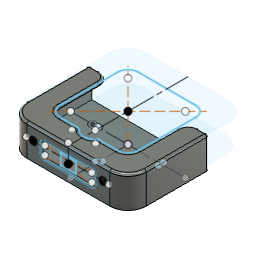
netgear-m5-wall-mount (Autodesk Fusion 360 design; units mm, degrees)
Autodesk Fusion 360 part; units mm, degrees
sketch "inner_space" plane through (0, 0, 0) normal (0, 1, 0) x (1, 0, 0)
  line L0 (-54.75, -54.75) -> (54.75, -54.75)
  line L1 (54.75, -54.75) -> (54.75, 54.75)
  line L2 (54.75, 54.75) -> (-54.75, 54.75)
  line L3 (-54.75, 54.75) -> (-54.75, -54.75)
  line L4 (-54.75, -54.75) -> (54.75, 54.75) construction
  line L5 (54.75, -54.75) -> (-54.75, 54.75) construction
  dimension "d21" = 109.5
  constraint horizontal L0
  constraint perpendicular L0 L1
  constraint parallel L0 L2
  constraint parallel L1 L3
  constraint coincident L4 origin
  constraint coincident L5 origin
  constraint equal L1 L2
  measures "d21" distance of L1.end L2.end
extrude "Extrude3" add sketch "inner_space" along normal blind 12.625 and the other way blind 12.625 makes body 1
fillet "Fillet2" radius 15 4 edges at (-54.75, 0, 54.75) (-54.75, 0, -54.75) (54.75, 0, 54.75) (54.75, 0, -54.75) on bodies 1
shell "Shell3" thickness 2.5 outward yes removed faces 0 bodies 1
sketch "bottom_ports" plane through (0, 0, 57.25) normal (0, 0, 1) x (1, 0, 0)
  line L0 (39.75, -15.125) -> (39.75, 15.125)
  line L1 (39.75, 15.125) -> (-39.75, 15.125)
  line L2 (-39.75, 15.125) -> (-39.75, -15.125)
  line L3 (-39.75, -15.125) -> (39.75, -15.125)
  line L4 (-7.2483, 5.7358) -> (7.2575, 5.7358)
  line L5 (7.2575, 5.7358) -> (7.2575, -4.8362)
  line L6 (7.2575, -4.8362) -> (-7.2483, -4.8362)
  line L7 (-7.2483, -4.8362) -> (-7.2483, 5.7358)
  line L8 (-40.1936, 2.575) -> (38.7277, 2.575) construction
  circle A0 centre (-33.5, 2.575) radius 3.3
  line L9 (0, 0) -> (0, 17.6954)
  circle A1 centre (33.5, 2.575) radius 3.3
  line L10 (22.5661, -8.0262) -> (-22.5661, -8.0262)
  line L11 (-26.5661, -4.0262) -> (-26.5661, 4.0262)
  line L12 (-22.5661, 8.0262) -> (22.5661, 8.0262)
  line L13 (26.5661, 4.0262) -> (26.5661, -4.0262)
  line L14 (26.5661, -8.0262) -> (-26.5661, 8.0262) construction
  line L15 (-26.5661, -8.0262) -> (26.5661, 8.0262) construction
  arc A2 (-22.5661, 8.0262) -> (-26.5661, 4.0262) centre (-22.5661, 4.0262) ccw
  arc A3 (-26.5661, -4.0262) -> (-22.5661, -8.0262) centre (-22.5661, -4.0262) ccw
  arc A4 (22.5661, -8.0262) -> (26.5661, -4.0262) centre (22.5661, -4.0262) ccw
  arc A5 (26.5661, 4.0262) -> (22.5661, 8.0262) centre (22.5661, 4.0262) ccw
  dimension "d41" = 6.6
  dimension "d45" = 4
  dimension "d91" = 33.5
  dimension "d94" = 17.7
  constraint horizontal L4
  constraint vertical L5
  constraint horizontal L6
  constraint vertical L7
  constraint perpendicular L0 L8
  constraint coincident L8 A0.centre
  constraint coincident L9.start origin
  constraint perpendicular L8 L9
  constraint symmetric A0 L9 A1
  constraint horizontal L10
  constraint perpendicular L10 L11
  constraint parallel L10 L12
  constraint parallel L11 L13
  constraint coincident L14 L9.start
  constraint coincident L15 L9.start
  constraint coincident L14.end L12
  constraint coincident L14.end L11
  constraint tangent L12 A2
  constraint tangent L11 A2
  constraint coincident L15.start L10
  constraint coincident L15.start L11
  constraint tangent L10 A3
  constraint tangent L11 A3
  constraint equal A2 A3
  constraint coincident L14.start L10
  constraint coincident L14.start L13
  constraint tangent L10 A4
  constraint tangent L13 A4
  constraint equal A2 A4
  constraint coincident L15.end L12
  constraint coincident L15.end L13
  constraint tangent L12 A5
  constraint tangent L13 A5
  constraint equal A2 A5
  measures "d41" diameter of A0
  measures "d45" radius of A2
  measures "d91" horizontal distance of A0.centre L9.end
  measures "d94" distance of L3 A0.centre
extrude "Extrude4" cut sketch "bottom_ports" against normal blind 10 contours L4 L5 L6 L7 | A0 | A1 | L10 L11 L12 L13 A2 A3 A4 A5 bodies 1
sketch "top_cutouts" plane through (0, 15.125, 0) normal (0, 1, 0) x (-1, 0, 0)
  arc A0 (-57.25, -39.75) -> (-39.75, -57.25) centre (-39.75, -39.75) ccw
  line L0 (-39.75, -57.25) -> (39.75, -57.25)
  arc A1 (39.75, -57.25) -> (57.25, -39.75) centre (39.75, -39.75) ccw
  line L1 (57.25, -39.75) -> (57.25, 39.75)
  arc A2 (57.25, 39.75) -> (39.75, 57.25) centre (39.75, 39.75) ccw
  line L2 (39.75, 57.25) -> (-39.75, 57.25)
  arc A3 (-39.75, 57.25) -> (-57.25, 39.75) centre (-39.75, 39.75) ccw
  line L3 (-57.25, 39.75) -> (-57.25, -39.75)
  line L4 (37.5, 27.5) -> (37.5, -27.5)
  line L5 (27.5, -37.5) -> (-27.5, -37.5)
  line L6 (-37.5, -27.5) -> (-37.5, 27.5)
  line L7 (-37.5, 37.5) -> (37.5, -37.5) construction
  line L8 (37.5, 37.5) -> (-37.5, -37.5) construction
  line L9 (0, -57.25) -> (0, 57.25)
  line L10 (-11.3811, 37.5) -> (-37.5, 37.5) construction
  line L11 (11.3811, 37.5) -> (27.5, 37.5)
  line L12 (-9.016, 37.5) -> (-27.5, 37.5)
  arc A4 (7.7879, 39.023) -> (-7.7879, 39.023) centre (0, 31.4868) ccw
  arc A5 (27.5, -37.5) -> (37.5, -27.5) centre (27.5, -27.5) ccw
  arc A6 (-37.5, -27.5) -> (-27.5, -37.5) centre (-27.5, -27.5) ccw
  arc A7 (-27.5, 37.5) -> (-37.5, 27.5) centre (-27.5, 27.5) ccw
  arc A8 (37.5, 27.5) -> (27.5, 37.5) centre (27.5, 27.5) ccw
  arc A9 (7.7879, 39.023) -> (11.3811, 37.5) centre (11.3811, 42.5) ccw
  arc A10 (-11.3811, 37.5) -> (-7.7879, 39.023) centre (-11.3811, 42.5) ccw
  dimension "d46" = 75
  dimension "d47" = 75
  dimension "d48" = 10
  dimension "d49" = 10
  dimension "d50" = 10
  dimension "d51" = 10
  dimension "d52" = 5
  dimension "d53" = 5
  constraint parallel L4 L6
  constraint coincident L7 origin
  constraint coincident L8 origin
  constraint midpoint L0 L9.start
  constraint midpoint L2 L9.end
  constraint perpendicular L6 L10
  constraint coincident L10 L12.start
  constraint coincident L7.end L5
  constraint coincident L7.end L4
  constraint tangent L5 A5
  constraint tangent L4 A5
  constraint coincident L8.end L5
  constraint coincident L8.end L6
  constraint tangent L5 A6
  constraint tangent L6 A6
  constraint coincident L7.start L12
  constraint coincident L7.start L6
  constraint tangent L12 A7
  constraint tangent L6 A7
  constraint coincident L8.start L4
  constraint coincident L8.start L11
  constraint tangent L4 A8
  constraint tangent L11 A8
  constraint tangent A4 A9
  constraint tangent L11 A9
  constraint tangent A4 A10
  constraint tangent L10 A10
  measures "d46" distance of L7.end L8.end
  measures "d47" distance of L8.start L7.end
  measures "d48" radius of A5
  measures "d49" radius of A6
  measures "d50" radius of A7
  measures "d51" radius of A8
  measures "d52" radius of A9
  measures "d53" radius of A10
extrude "Extrude5" cut sketch "top_cutouts" against normal blind 5 contours L4 L5 L9 L11 A4 A5 A8 A9 | L5 L6 L9 L12 A4 A6 A7 A10 bodies 1
sketch "mounting_holes" plane through (0, -12.625, 0) normal (0, 1, 0) x (-1, 0, 0)
  arc A0 (-54.75, -39.75) -> (-39.75, -54.75) centre (-39.75, -39.75) ccw
  line L0 (-39.75, -54.75) -> (39.75, -54.75)
  arc A1 (39.75, -54.75) -> (54.75, -39.75) centre (39.75, -39.75) ccw
  line L1 (54.75, -39.75) -> (54.75, 39.75)
  arc A2 (54.75, 39.75) -> (39.75, 54.75) centre (39.75, 39.75) ccw
  line L2 (39.75, 54.75) -> (-39.75, 54.75)
  arc A3 (-39.75, 54.75) -> (-54.75, 39.75) centre (-39.75, 39.75) ccw
  line L3 (-54.75, 39.75) -> (-54.75, -39.75)
  line L4 (0, 0) -> (-54.9589, 0)
  line L5 (0, 0) -> (0, 55.0492)
  line L6 (0, 0) -> (54.9589, 0)
  line L7 (33.9306, -2) -> (28.9306, -2)
  line L8 (33.9306, 2) -> (28.9306, 2)
  arc A4 (33.9306, -2) -> (33.9306, 2) centre (33.9306, 0) ccw
  arc A5 (28.9306, 2) -> (28.9306, -2) centre (28.9306, 0) ccw
  line L9 (-29.8211, -2.2468) -> (-29.8211, 2.7532)
  arc A6 (-33.8211, -2.2468) -> (-29.8211, -2.2468) centre (-31.8211, -2.2468) ccw
  line L10 (-33.8211, -2.2468) -> (-33.8211, 2.7532)
  arc A7 (-29.8211, 2.7532) -> (-33.8211, 2.7532) centre (-31.8211, 2.7532) ccw
  line L11 (0.4454, 30.8513) -> (-3.0902, 27.3157)
  arc A8 (3.2738, 28.0228) -> (0.4454, 30.8513) centre (1.8596, 29.437) ccw
  line L12 (3.2738, 28.0228) -> (-0.2617, 24.4873)
  arc A9 (-3.0902, 27.3157) -> (-0.2617, 24.4873) centre (-1.676, 25.9015) ccw
  point P0 (33.9306, 0)
  dimension "d56" = 4
  dimension "d57" = 4
  dimension "d58" = 4
  dimension "d59" = 4
  dimension "d60" = 4
  dimension "d61" = 4
  constraint coincident L4.start L5.start
  constraint perpendicular L3 L4
  constraint perpendicular L2 L5
  constraint symmetric L4.start L5 L6.start
  constraint symmetric L4.end L5 L6.end
  constraint coincident L6 P0
  constraint tangent L7 A5
  constraint tangent L8 A5
  constraint tangent L7 A4
  constraint tangent L8 A4
  constraint tangent L10 A7
  constraint tangent L9 A7
  constraint tangent A6 L10
  constraint tangent L9 A6
  constraint tangent L12 A9
  constraint tangent L11 A9
  constraint tangent A8 L12
  constraint tangent L11 A8
  measures "d56" diameter of A4
  measures "d57" diameter of A5
  measures "d58" diameter of A6
  measures "d59" diameter of A7
  measures "d60" diameter of A8
  measures "d61" diameter of A9
extrude "Extrude6" cut sketch "mounting_holes" against normal blind 8 contours L4 L9 L10 A7 | L4 L9 A6 L10 | L6 L7 A4 A5 | L6 L8 A4 A5 | L5 L11 A8 L12 | L5 L11 L12 A9 bodies 1
chamfer "Chamfer1" distance 1.5 angle 45 12 edges at (-31.4306, -12.625, -2) (-26.9306, -12.625, 0) (-31.4306, -12.625, 2) (-35.9306, -12.625, 0) (3.0902, -12.625, 24.4873) (1.3224, -12.625, 29.0835) (-3.2738, -12.625, 30.8513) (-1.506, -12.625, 26.2551) (31.8211, -12.625, 4.7532) (29.8211, -12.625, 0.2532) (31.8211, -12.625, -4.2468) (33.8211, -12.625, 0.2532) on bodies 1
ref_plane "WorkPlane1" through (0, 0, -20) normal (0, 0, 1) x (1, 0, 0)
split "Split2" by plane through (0, 0, -20) normal (0, 0, 1) bodies 1 makes body 2 at (-31.6796, -15.125, 23.7041)
fillet "Fillet3" radius 10 2 edges at (-37.5, 13.875, -20) (37.5, 13.875, -20) on bodies 2
sketch "Sketch12" plane through (0, 0, 54.75) normal (0, 0, -1) x (-1, 0, 0)
  circle A0 centre (33.5, 2.575) radius 3.3
  circle A1 centre (-33.5, 2.575) radius 3.3
  line L0 (-26.5661, -4.0262) -> (-26.5661, 4.0262)
  arc A2 (-22.5661, 8.0262) -> (-26.5661, 4.0262) centre (-22.5661, 4.0262) ccw
  line L1 (-22.5661, 8.0262) -> (22.5661, 8.0262)
  arc A3 (26.5661, 4.0262) -> (22.5661, 8.0262) centre (22.5661, 4.0262) ccw
  line L2 (26.5661, 4.0262) -> (26.5661, -4.0262)
  arc A4 (22.5661, -8.0262) -> (26.5661, -4.0262) centre (22.5661, -4.0262) ccw
  line L3 (22.5661, -8.0262) -> (-22.5661, -8.0262)
  arc A5 (-26.5661, -4.0262) -> (-22.5661, -8.0262) centre (-22.5661, -4.0262) ccw
  line L4 (-39.75, 12.625) -> (-39.75, -12.625)
  line L5 (-39.75, -12.625) -> (39.75, -12.625)
  line L6 (39.75, -12.625) -> (39.75, 12.625)
  line L7 (39.75, 12.625) -> (-39.75, 12.625)
  circle A6 centre (33.5, 2.575) radius 5
  line L8 (0, 0) -> (0, 17.6781)
  circle A7 centre (-33.5, 2.575) radius 5
  dimension "d68" = 10
  constraint concentric A0 A6
  constraint coincident L8.start origin
  constraint perpendicular L7 L8
  constraint symmetric A6 L8 A7
  measures "d68" diameter of A6
extrude "Extrude7" cut sketch "Sketch12" against normal blind 1.5 contours A6 | A7 bodies 2
fillet "Fillet12" radius 3 5 edges at (-54.75, 12.625, 9.875) (-50.3566, 12.625, 50.3566) (0, 12.625, 54.75) (50.3566, 12.625, 50.3566) (54.75, 12.625, 9.875) on bodies 2
fillet "Fillet13" radius 2 5 edges at (-57.25, 15.125, 9.875) (-52.1244, 15.125, 52.1244) (0, 15.125, 57.25) (52.1244, 15.125, 52.1244) (57.25, 15.125, 9.875) 1 faces at (-50.6667, 15.125, 15.75) on bodies 2
fillet "Fillet14" radius 2 4 edges at (57.25, -1, -20) (56.6642, 14.5392, -19.4142) (-56.6642, 14.5392, -19.4142) (-57.25, -1, -20) on bodies 2
hidden bodies 1
equation "d21 = 105.5 mm + ( 2 * 2 ) * 1 mm"
equation "d91 = ( 67 / 2 ) * 1 mm"
equation "d94 = 2.5 mm + 2 mm + 13.2 mm"
named bodies: "case_lower"
